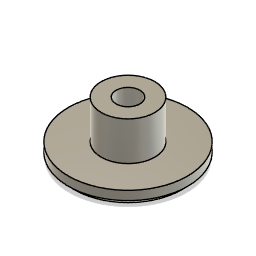
タイヤ+固定具 (Autodesk Fusion 360 archive; units mm, degrees)
design "モーター_ホイール　固定具"
Autodesk Fusion 360 part; units mm, degrees
sketch "スケッチ1" plane through (0, 0, 0) normal (0, 1, 0) x (1, 0, 0)
  circle A0 centre (0, 0) radius 10
  dimension "d1" = 20
  constraint coincident A0.centre origin
  measures "d1" diameter of A0
extrude "押し出し1" add sketch "スケッチ1" along normal blind 2.5
sketch "スケッチ2" plane through (0, 2.5, 0) normal (0, 1, 0) x (-1, 0, 0)
  circle A0 centre (0, 0) radius 10
  circle A1 centre (0, 0) radius 4.5
  dimension "d4" = 9
  constraint coincident A0.centre A1.centre
  measures "d4" diameter of A1
extrude "押し出し2" add sketch "スケッチ2" along normal blind 6.5 contours A1
sketch "スケッチ4" plane through (0, 0, 0) normal (0, -1, 0) x (1, 0, 0)
  circle A0 centre (0, 0) radius 2
  circle A1 centre (0, 0) radius 10
  dimension "d9" = 4
  constraint coincident A0.centre A1.centre
  measures "d9" diameter of A0
extrude "押し出し3" cut sketch "スケッチ4" against normal blind 16 contours A0
sketch "スケッチ5" plane through (0, 0, 0) normal (0, 0, 1) x (1, 0, 0)
  line L0 (10, 0) -> (10, 1)
  line L1 (10, 1) -> (9, 0)
  line L2 (9, 0) -> (10, 0)
  constraint vertical L0
  constraint perpendicular L0 L2
revolve "回転2" cut sketch "スケッチ5" angle 360 about axis through (0, 1.75, 0) along (0, 1, 0)
